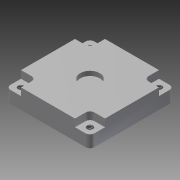
# Autodesk Inventor part: stepper_bottom_28
Saved by Autodesk Inventor 2013 (Build 170138000, 138)
## iProperties
Shininess: 50.0
Created: 2013-02-12
Part Number: stepper_bottom_28
Document SubType Name: Modeling
Designer: Noa Izumi
Material: Default
Density: 1 g/cm^3
Density: 0.0
Volumn: 0.0
Area: 0.0
PropertySet Name: Model Information
Control State: 0
Master: False
Checked Out: False
Author: Noa Izumi
Autodesk Inventor part; units mm, degrees
ref_plane "YZ Plane" through (0, 0, 0) normal (1, 0, 0) x (0, 1, 0)
ref_plane "XZ Plane" through (0, 0, 0) normal (0, 1, 0) x (-1, 0, 0)
ref_plane "XY Plane" through (0, 0, 0) normal (0, 0, 1) x (1, 0, 0)
sketch "Sketch1" plane through (0, 0, 0) normal (0, 0, 1) x (1, 0, 0)
  line L0 (0, 0) -> (28, 0)
  line L1 (28, 0) -> (28, 28)
  line L2 (28, 28) -> (0, 28)
  line L3 (0, 28) -> (0, 0)
  dimension "d0" = 28
  dimension "d1" = 28
  constraints: 8 end point, 2 parallel, 1 horizontal, 1 perpendicular
  measures "d0" distance of L2.end L0.start
  measures "d1" distance of L0.start L0.end
extrude "Extrusion1" add sketch "Sketch1" along normal blind 6.5
sketch "Sketch6" plane through (0, 0, 6.5) normal (0, 0, 1) x (1, 0, 0)
  line L0 (0, 0) -> (5, 0)
  line L1 (5, 0) -> (5, 5)
  line L2 (5, 5) -> (0, 5)
  line L3 (0, 5) -> (0, 0)
  line L4 (23, 5) -> (28, 5)
  line L5 (28, 5) -> (28, 0)
  line L6 (28, 0) -> (23, 0)
  line L7 (23, 0) -> (23, 5)
  line L8 (0, 28) -> (5, 28)
  line L9 (5, 28) -> (5, 23)
  line L10 (5, 23) -> (0, 23)
  line L11 (0, 23) -> (0, 28)
  line L12 (28, 28) -> (23, 28)
  line L13 (23, 28) -> (23, 23)
  line L14 (23, 23) -> (28, 23)
  line L15 (28, 23) -> (28, 28)
  dimension "d28" = 5
  dimension "d29" = 5
  dimension "d30" = 5
  dimension "d31" = 5
  dimension "d32" = 5
  constraints: 32 end point, 8 parallel, 4 horizontal, 4 perpendicular
  measures "d28" distance of L2.end L0.start
  measures "d29" distance of L1.end L2.end
  measures "d30" distance of L5.end L6.end
  measures "d31" distance of L6.end L4.start
  measures "d32" distance of L8.end L9.end
extrude "Extrusion4" cut sketch "Sketch6" against normal blind 2.5
fillet "Fillet2" radius 1.5 8 edges at (0, 0, 2) (5, 5, 5.25) (0, 28, 2) (5, 23, 5.25) (23, 23, 5.25) (28, 28, 2) (23, 5, 5.25) (28, 0, 2)
sketch "Sketch7" plane through (0, 0, 4) normal (0, 0, 1) x (1, 0, 0)
  line L0 (0, 23) -> (0, 26.5) projected
  line L1 (1.5, 28) -> (5, 28) projected
  line L2 (5, 0) -> (1.5, 0) projected
  line L3 (28, 23) -> (28, 5) projected
  line L4 (0, 1.5) -> (0, 5) projected
  line L5 (5, 28) -> (23, 28) projected
  line L6 (23, 0) -> (5, 0) projected
  point P0 (2.5, 25.5)
  point P1 (2.5, 2.5)
  point P2 (25.5, 25.5)
  point P3 (25.5, 2.5)
  dimension "d36" = 2.5
  dimension "d37" = 2.5
  dimension "d38" = 2.5
  dimension "d39" = 2.5
  dimension "d52" = 2.5
  dimension "d53" = 2.5
  dimension "d54" = 2.5
  dimension "d55" = 2.5
  measures "d36" distance from line of point (2.5, 25.5) L1
  measures "d37" distance from line of L0 point (2.5, 25.5)
  measures "d38" distance from line of point (2.5, 2.5) L2
  measures "d39" distance from line of L3 point (25.5, 25.5)
  measures "d52" distance from line of L4 point (2.5, 2.5)
  measures "d53" distance from line of point (25.5, 25.5) L5
  measures "d54" distance from line of point (25.5, 2.5) L3
  measures "d55" distance from line of point (25.5, 2.5) L6
hole "Hole2" at (2.5, 25.5, 4) at (2.5, 2.5, 4) at (25.5, 25.5, 4) at (25.5, 2.5, 4) direction (0, 0, -1) diameter 2.013 end through all thread size "M2.5x0.45" class "6H" standard "ANSI Metric M Profile"
sketch "Sketch8" plane through (0, 0, 6.5) normal (0, 0, 1) x (1, 0, 0)
  line L0 (5, 28) -> (23, 28) projected
  line L1 (0, 5) -> (0, 23) projected
  circle A0 centre (14, 14) radius 3.25
  dimension "d47" = 6.5
  dimension "d48" = 14
  dimension "d49" = 14
  constraints: 1 centre point
  measures "d47" diameter of A0
  measures "d48" distance from line of L1 A0.centre
  measures "d49" distance from line of L0 A0.centre
extrude "Extrusion5" cut sketch "Sketch8" against normal blind 1.5
